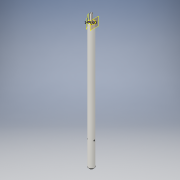
# Autodesk Inventor part: Welle
Saved by Autodesk Inventor 2018 (Build 220112000, 112)
## iProperties
Created: 2017-10-13
Part Number: Welle
Material: Stahl
Document SubType Name: Modeling
Designer: Dominik
Density: 7.85 g/cm^3
Appearance: Platte
Mass: 457.438 g
Surface Area: 162.584 cm^2
Volume: 58.2723 cm^3
Author: Dominik
Autodesk Inventor part; units mm, degrees
ref_plane "YZ Plane" through (0, 0, 0) normal (1, 0, 0) x (0, 1, 0)
ref_plane "XZ Plane" through (0, 0, 0) normal (0, 1, 0) x (-1, 0, 0)
ref_plane "XY Plane" through (0, 0, 0) normal (0, 0, 1) x (1, 0, 0)
sketch "Skizze1" plane through (0, 0, 0) normal (0, 0, 1) x (1, 0, 0)
  circle A0 centre (0, 0) radius 7.5
  dimension "d0" = 15
  constraints: 1 centre point, 1 coincident
  measures "d0" diameter of A0
extrude "Extrusion1" add sketch "Skizze1" along normal blind 330
sketch "Skizze2" plane through (0, 0, 330) normal (0, 0, 1) x (1, 0, 0)
  point P0 (0, 0)
sketch "Skizze5" plane through (0, 0, 330) normal (0, 0, 1) x (1, 0, 0)
  line L0 (0, 0) -> (0, 2)
  line L1 (0, 2) -> (2, 2)
  line L2 (2, 2) -> (2, -2)
  line L3 (2, -2) -> (-2, -2)
  line L4 (-2, -2) -> (-2, 2)
  line L5 (-2, 2) -> (0, 2)
  dimension "d8" = 2
  dimension "d9" = 2
  dimension "d10" = 4
  dimension "d11" = 4
  dimension "d12" = 4
  constraints: 12 end point, 3 perpendicular, 1 point on line, 1 vertical
  measures "d8" distance of L0.start L0.end
  measures "d9" distance of L0.end L1.end
  measures "d10" distance of L1.end L2.end
  measures "d11" distance of L2.end L3.end
  measures "d12" distance of L3.end L4.end
extrude "Extrusion4" add sketch "Skizze5" along normal blind 20
sketch "Skizze6" plane through (0, 0, 330) normal (0, 0, 1) x (1, 0, 0)
  line L0 (0, 0) -> (-6.0676, -4.4084)
  circle A0 centre (0, 0) radius 7.5 projected
  line L1 (0, 0) -> (7.5, 0) construction
  line L2 (0, 0) -> (7.5, 0)
  line L3 (2, -2) -> (2, 2) projected
  dimension "d15" = 144
  constraints: 6 end point, 1 equal length, 1 horizontal, 1 perpendicular, 2 other
  measures "d15" angle of L0 L1
ref_plane "Arbeitsebene1" through (-6.0676, -4.4084, 330) normal (-0.809017, -0.5877853, 0) x (0.5877853, -0.809017, 0)
sketch "Skizze7" plane through (-6.0676, -4.4084, 330) normal (-0.809017, -0.5877853, 0) x (0.5877853, -0.809017, 0)
  line L0 (7.5, 0) -> (-7.5, 0) projected
  line L1 (0, 0) -> (0, -265)
  line L2 (-15, -336) -> (15, -336) projected
  point P0 (0, -330)
  dimension "d16" = 265
  constraints: 2 end point, 1 midpoint, 1 perpendicular
  measures "d16" distance of L1.start L1.end
hole "Bohrung1" at (-6.0676, -4.4084, 65) direction (0.809017, 0.5877853, 0) diameter 3.2 depth 4 tip angle 118
ref_plane "Arbeitsebene2" through (7.5, 0, 330) normal (1, 0, 0) x (0, 1, 0)
sketch "Skizze8" plane through (7.5, 0, 330) normal (1, 0, 0) x (0, 1, 0)
  line L0 (7.5, 0) -> (-7.5, 0) projected
  line L1 (0, 0) -> (0, -265)
  point P0 (0, -330)
  dimension "d24" = 265
  constraints: 2 end point, 1 midpoint, 1 vertical
  measures "d24" distance of L1.start L1.end
hole "Bohrung2" at (7.5, 0, 65) direction (-1, 0, 0) diameter 3.2 depth 4 tip angle 118
sketch "Skizze9" plane through (0, 0, 0) normal (0, 0, -1) x (-1, 0, 0)
  circle A0 centre (0, 0) radius 5
  circle A1 centre (0, 0) radius 7.5
  dimension "d32" = 10
  constraints: 2 centre point, 2 coincident
  measures "d32" diameter of A0
extrude "Extrusion5" cut sketch "Skizze9" against normal blind 3
